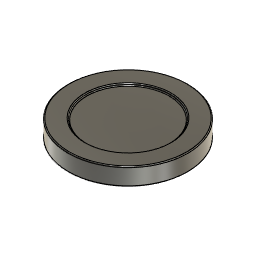
puck2 v2 (Autodesk Fusion 360 design; units mm, degrees)
Autodesk Fusion 360 part; units mm, degrees
sketch "Skizze1" plane through (0, 0, 0) normal (0, 0, 1) x (1, 0, 0)
  circle A0 centre (0, 0) radius 34
  dimension "d1" = 68
  constraint coincident A0.centre origin
  measures "d1" diameter of A0
extrude "Extrusion1" add sketch "Skizze1" along normal blind 10
sketch "Skizze2" plane through (0, 0, 10) normal (0, 0, 1) x (-1, 0, 0)
  circle A0 centre (0, 0) radius 34
  circle A1 centre (0, 0) radius 24
  dimension "d4" = 48
  constraint coincident A0.centre A1.centre
  measures "d4" diameter of A1
extrude "Extrusion2" cut sketch "Skizze2" against normal blind 1 contours A1
sketch "Skizze3" plane through (0, 0, 0) normal (0, 0, -1) x (1, 0, 0)
  circle A0 centre (0, 0) radius 34
  circle A1 centre (0, 0) radius 24
  dimension "d7" = 48
  constraint coincident A0.centre A1.centre
  measures "d7" diameter of A1
extrude "Extrusion3" cut sketch "Skizze3" against normal blind 1 contours A1
fillet "Abrundung1" radius 0.5 6 edges at (22.3759, -8.6788, 9) (-31.6991, -12.2949, 10) (-31.6991, -12.2949, 0) (-22.3759, -8.6788, 0) (-22.3759, -8.6788, 1) (22.3759, -8.6788, 10)
